Autodesk Fusion 360 part; units mm, degrees
(part 2 of 2)
sketch "Access Holes (Front)" plane through (-47, 0, 0) normal (1, 0, 0) x (0, 1, 0)
  line L0 (-30, 10) -> (30, 10)
  line L1 (30, 10) -> (30, 28)
  line L2 (30, 28) -> (-30, 28)
  line L3 (-30, 28) -> (-30, 10)
  line L4 (-18, 28) -> (-18, 10)
  line L5 (-9, 10) -> (-27, 10)
  line L6 (9, 28) -> (-7.0946, 28)
  line L7 (-7, 10) -> (9.0946, 10)
  line L8 (9, 28) -> (-7, 10) construction
  line L9 (-27, 10) -> (-9, 10)
  line L10 (-9, 10) -> (-9, 28)
  line L11 (-9, 28) -> (-27, 28)
  line L12 (-27, 28) -> (-27, 10)
  line L13 (-7, 10) -> (9, 10)
  line L14 (9, 10) -> (9, 28)
  line L15 (9, 28) -> (-7, 28)
  line L16 (-7, 28) -> (-7, 10)
  line L17 (11, 10) -> (27, 10)
  line L18 (27, 10) -> (27, 28)
  line L19 (27, 28) -> (11, 28)
  line L20 (11, 28) -> (11, 10)
  line L21 (30, 10) -> (-30, 10)
  line L22 (-13.2569, 0) -> (-15.855, 0)
  line L23 (-15.855, 0) -> (-18.4531, 0)
  line L24 (-18.4531, 0) -> (-15.855, 0)
  line L25 (-15.855, 0) -> (-13.2569, 0)
  line L26 (-15.4901, 0) -> (-12.892, 0)
  line L27 (-12.892, 0) -> (-10.2939, 0)
  line L28 (-10.2939, 0) -> (-12.892, 0)
  line L29 (-12.892, 0) -> (-15.4901, 0)
  line L30 (-7.0879, 0) -> (-9.686, 0)
  line L31 (-9.686, 0) -> (-12.2841, 0)
  line L32 (-12.2841, 0) -> (-9.686, 0)
  line L33 (-9.686, 0) -> (-7.0879, 0)
  line L34 (-21.6861, 0) -> (-19.088, 0)
  line L35 (-19.088, 0) -> (-16.4899, 0)
  line L36 (-16.4899, 0) -> (-19.088, 0)
  line L37 (-19.088, 0) -> (-21.6861, 0)
  line L38 (-15.4901, 0) -> (-12.892, 0)
  line L39 (-12.892, 0) -> (-10.2939, 0)
  line L40 (-10.2939, 0) -> (-12.892, 0)
  line L41 (-12.892, 0) -> (-15.4901, 0)
  line L42 (-9.2941, 0) -> (-6.696, 0)
  line L43 (-6.696, 0) -> (-4.0979, 0)
  line L44 (-4.0979, 0) -> (-6.696, 0)
  line L45 (-6.696, 0) -> (-9.2941, 0)
  line L46 (-0.5, 0) -> (2.0981, 0)
  line L47 (2.0981, 0) -> (-0.5, 0)
  line L48 (-0.5, 0) -> (-3.0981, 0)
  line L49 (-3.0981, 0) -> (-0.5, 0)
  line L50 (-9.2941, 0) -> (-6.696, 0)
  line L51 (-6.696, 0) -> (-4.0979, 0)
  line L52 (-4.0979, 0) -> (-6.696, 0)
  line L53 (-6.696, 0) -> (-9.2941, 0)
  line L54 (-7.0879, 0) -> (-9.686, 0)
  line L55 (-9.686, 0) -> (-12.2841, 0)
  line L56 (-12.2841, 0) -> (-9.686, 0)
  line L57 (-9.686, 0) -> (-7.0879, 0)
  line L58 (-0.9189, 0) -> (-3.517, 0)
  line L59 (-3.517, 0) -> (-6.1151, 0)
  line L60 (-6.1151, 0) -> (-3.517, 0)
  line L61 (-3.517, 0) -> (-0.9189, 0)
  line L62 (5.2501, 0) -> (2.652, 0)
  line L63 (2.652, 0) -> (0.0539, 0)
  line L64 (0.0539, 0) -> (2.652, 0)
  line L65 (2.652, 0) -> (5.2501, 0)
  line L66 (11.4191, 0) -> (8.821, 0)
  line L67 (8.821, 0) -> (6.2229, 0)
  line L68 (6.2229, 0) -> (8.821, 0)
  line L69 (8.821, 0) -> (11.4191, 0)
  line L70 (5.696, 0) -> (8.2941, 0)
  line L71 (8.2941, 0) -> (5.696, 0)
  line L72 (5.696, 0) -> (3.0979, 0)
  line L73 (3.0979, 0) -> (5.696, 0)
  line L74 (18.088, 0) -> (15.4899, 0)
  line L75 (15.4899, 0) -> (18.088, 0)
  line L76 (18.088, 0) -> (20.6861, 0)
  line L77 (20.6861, 0) -> (18.088, 0)
  line L78 (11.892, 0) -> (14.4901, 0)
  line L79 (14.4901, 0) -> (11.892, 0)
  line L80 (11.892, 0) -> (9.2939, 0)
  line L81 (9.2939, 0) -> (11.892, 0)
  line L82 (-0.5, 0) -> (2.0981, 0)
  line L83 (2.0981, 0) -> (-0.5, 0)
  line L84 (-0.5, 0) -> (-3.0981, 0)
  line L85 (-3.0981, 0) -> (-0.5, 0)
  line L86 (11.4191, 0) -> (8.821, 0)
  line L87 (8.821, 0) -> (6.2229, 0)
  line L88 (6.2229, 0) -> (8.821, 0)
  line L89 (8.821, 0) -> (11.4191, 0)
  line L90 (11.4191, 0) -> (8.821, 0)
  line L91 (8.821, 0) -> (6.2229, 0)
  line L92 (6.2229, 0) -> (8.821, 0)
  line L93 (8.821, 0) -> (11.4191, 0)
  line L94 (20.6861, 0) -> (18.088, 0)
  line L95 (18.088, 0) -> (15.4899, 0)
  line L96 (15.4899, 0) -> (18.088, 0)
  line L97 (18.088, 0) -> (20.6861, 0)
  line L98 (20.6861, 0) -> (18.088, 0)
  line L99 (18.088, 0) -> (15.4899, 0)
  line L100 (15.4899, 0) -> (18.088, 0)
  line L101 (18.088, 0) -> (20.6861, 0)
  line L102 (17.5881, 0) -> (14.99, 0)
  line L103 (14.99, 0) -> (12.3919, 0)
  line L104 (12.3919, 0) -> (14.99, 0)
  line L105 (14.99, 0) -> (17.5881, 0)
  line L106 (11.892, 0) -> (14.4901, 0)
  line L107 (14.4901, 0) -> (11.892, 0)
  line L108 (11.892, 0) -> (9.2939, 0)
  line L109 (9.2939, 0) -> (11.892, 0)
  line L110 (5.2501, 0) -> (2.652, 0)
  line L111 (2.652, 0) -> (0.0539, 0)
  line L112 (0.0539, 0) -> (2.652, 0)
  line L113 (2.652, 0) -> (5.2501, 0)
  line L114 (5.2501, 0) -> (2.652, 0)
  line L115 (2.652, 0) -> (0.0539, 0)
  line L116 (0.0539, 0) -> (2.652, 0)
  line L117 (2.652, 0) -> (5.2501, 0)
  line L118 (17.5881, 0) -> (14.99, 0)
  line L119 (14.99, 0) -> (12.3919, 0)
  line L120 (12.3919, 0) -> (14.99, 0)
  line L121 (14.99, 0) -> (17.5881, 0)
  line L122 (9.2939, 0) -> (11.892, 0)
  line L123 (11.892, 0) -> (14.4901, 0)
  line L124 (14.4901, 0) -> (11.892, 0)
  line L125 (11.892, 0) -> (9.2939, 0)
  line L126 (11.4191, 0) -> (8.821, 0)
  line L127 (8.821, 0) -> (6.2229, 0)
  line L128 (6.2229, 0) -> (8.821, 0)
  line L129 (8.821, 0) -> (11.4191, 0)
  line L130 (5.2501, 0) -> (2.652, 0)
  line L131 (2.652, 0) -> (0.0539, 0)
  line L132 (0.0539, 0) -> (2.652, 0)
  line L133 (2.652, 0) -> (5.2501, 0)
  line L134 (-0.9189, 0) -> (-3.517, 0)
  line L135 (-3.517, 0) -> (-6.1151, 0)
  line L136 (-6.1151, 0) -> (-3.517, 0)
  line L137 (-3.517, 0) -> (-0.9189, 0)
  line L138 (-7.0879, 0) -> (-9.686, 0)
  line L139 (-9.686, 0) -> (-12.2841, 0)
  line L140 (-12.2841, 0) -> (-9.686, 0)
  line L141 (-9.686, 0) -> (-7.0879, 0)
  line L142 (3.0979, 0) -> (5.696, 0)
  line L143 (5.696, 0) -> (8.2941, 0)
  line L144 (8.2941, 0) -> (5.696, 0)
  line L145 (5.696, 0) -> (3.0979, 0)
  line L146 (-0.9189, 0) -> (-3.517, 0)
  line L147 (-3.517, 0) -> (-6.1151, 0)
  line L148 (-6.1151, 0) -> (-3.517, 0)
  line L149 (-3.517, 0) -> (-0.9189, 0)
  line L150 (-9.2941, 0) -> (-6.696, 0)
  line L151 (-6.696, 0) -> (-4.0979, 0)
  line L152 (-4.0979, 0) -> (-6.696, 0)
  line L153 (-6.696, 0) -> (-9.2941, 0)
  line L154 (-15.4901, 0) -> (-12.892, 0)
  line L155 (-12.892, 0) -> (-10.2939, 0)
  line L156 (-10.2939, 0) -> (-12.892, 0)
  line L157 (-12.892, 0) -> (-15.4901, 0)
  line L158 (-21.6861, 0) -> (-19.088, 0)
  line L159 (-19.088, 0) -> (-16.4899, 0)
  line L160 (-16.4899, 0) -> (-19.088, 0)
  line L161 (-19.088, 0) -> (-21.6861, 0)
  line L162 (-15.4901, 0) -> (-12.892, 0)
  line L163 (-12.892, 0) -> (-10.2939, 0)
  line L164 (-10.2939, 0) -> (-12.892, 0)
  line L165 (-12.892, 0) -> (-15.4901, 0)
  line L166 (-15.4901, 0) -> (-12.892, 0)
  line L167 (-12.892, 0) -> (-10.2939, 0)
  line L168 (-10.2939, 0) -> (-12.892, 0)
  line L169 (-12.892, 0) -> (-15.4901, 0)
  line L170 (-21.6861, 0) -> (-19.088, 0)
  line L171 (-19.088, 0) -> (-16.4899, 0)
  line L172 (-16.4899, 0) -> (-19.088, 0)
  line L173 (-19.088, 0) -> (-21.6861, 0)
  line L174 (-21.6861, 0) -> (-19.088, 0)
  line L175 (-19.088, 0) -> (-16.4899, 0)
  line L176 (-16.4899, 0) -> (-19.088, 0)
  line L177 (-19.088, 0) -> (-21.6861, 0)
  line L178 (-21.6861, 0) -> (-19.088, 0)
  line L179 (-19.088, 0) -> (-16.4899, 0)
  line L180 (-16.4899, 0) -> (-19.088, 0)
  line L181 (-19.088, 0) -> (-21.6861, 0)
  line L182 (-13.2569, 0) -> (-15.855, 0)
  line L183 (-15.855, 0) -> (-18.4531, 0)
  line L184 (-18.4531, 0) -> (-15.855, 0)
  line L185 (-15.855, 0) -> (-13.2569, 0)
  line L186 (-9.2941, 0) -> (-6.696, 0)
  line L187 (-6.696, 0) -> (-4.0979, 0)
  line L188 (-4.0979, 0) -> (-6.696, 0)
  line L189 (-6.696, 0) -> (-9.2941, 0)
  line L190 (-15.4901, 0) -> (-12.892, 0)
  line L191 (-12.892, 0) -> (-10.2939, 0)
  line L192 (-10.2939, 0) -> (-12.892, 0)
  line L193 (-12.892, 0) -> (-15.4901, 0)
  line L194 (-13.2569, 0) -> (-15.855, 0)
  line L195 (-15.855, 0) -> (-18.4531, 0)
  line L196 (-18.4531, 0) -> (-15.855, 0)
  line L197 (-15.855, 0) -> (-13.2569, 0)
  line L198 (-7.0879, 0) -> (-9.686, 0)
  line L199 (-9.686, 0) -> (-12.2841, 0)
  line L200 (-12.2841, 0) -> (-9.686, 0)
  line L201 (-9.686, 0) -> (-7.0879, 0)
  line L202 (-0.9189, 0) -> (-3.517, 0)
  line L203 (-3.517, 0) -> (-6.1151, 0)
  line L204 (-6.1151, 0) -> (-3.517, 0)
  line L205 (-3.517, 0) -> (-0.9189, 0)
  line L206 (5.2501, 0) -> (2.652, 0)
  line L207 (2.652, 0) -> (0.0539, 0)
  line L208 (0.0539, 0) -> (2.652, 0)
  line L209 (2.652, 0) -> (5.2501, 0)
  line L210 (-0.9189, 0) -> (-3.517, 0)
  line L211 (-3.517, 0) -> (-6.1151, 0)
  line L212 (-6.1151, 0) -> (-3.517, 0)
  line L213 (-3.517, 0) -> (-0.9189, 0)
  line L214 (-9.2941, 0) -> (-6.696, 0)
  line L215 (-6.696, 0) -> (-4.0979, 0)
  line L216 (-4.0979, 0) -> (-6.696, 0)
  line L217 (-6.696, 0) -> (-9.2941, 0)
  line L218 (-0.5, 0) -> (2.0981, 0)
  line L219 (2.0981, 0) -> (-0.5, 0)
  line L220 (-0.5, 0) -> (-3.0981, 0)
  line L221 (-3.0981, 0) -> (-0.5, 0)
  line L222 (5.696, 0) -> (8.2941, 0)
  line L223 (8.2941, 0) -> (5.696, 0)
  line L224 (5.696, 0) -> (3.0979, 0)
  line L225 (3.0979, 0) -> (5.696, 0)
  line L226 (11.892, 0) -> (14.4901, 0)
  line L227 (14.4901, 0) -> (11.892, 0)
  line L228 (11.892, 0) -> (9.2939, 0)
  line L229 (9.2939, 0) -> (11.892, 0)
  line L230 (12.3919, 0) -> (14.99, 0)
  line L231 (14.99, 0) -> (17.5881, 0)
  line L232 (17.5881, 0) -> (14.99, 0)
  line L233 (14.99, 0) -> (12.3919, 0)
  line L234 (17.5881, 0) -> (14.99, 0)
  line L235 (14.99, 0) -> (12.3919, 0)
  line L236 (12.3919, 0) -> (14.99, 0)
  line L237 (14.99, 0) -> (17.5881, 0)
  line L238 (5.696, 0) -> (8.2941, 0)
  line L239 (8.2941, 0) -> (5.696, 0)
  line L240 (5.696, 0) -> (3.0979, 0)
  line L241 (3.0979, 0) -> (5.696, 0)
  line L242 (17.5881, 0) -> (14.99, 0)
  line L243 (14.99, 0) -> (12.3919, 0)
  line L244 (12.3919, 0) -> (14.99, 0)
  line L245 (14.99, 0) -> (17.5881, 0)
  line L246 (17.5881, 0) -> (14.99, 0)
  line L247 (14.99, 0) -> (12.3919, 0)
  line L248 (12.3919, 0) -> (14.99, 0)
  line L249 (14.99, 0) -> (17.5881, 0)
  line L250 (20.6861, 0) -> (18.088, 0)
  line L251 (18.088, 0) -> (15.4899, 0)
  line L252 (15.4899, 0) -> (18.088, 0)
  line L253 (18.088, 0) -> (20.6861, 0)
  line L254 (20.6861, 0) -> (18.088, 0)
  line L255 (18.088, 0) -> (15.4899, 0)
  line L256 (15.4899, 0) -> (18.088, 0)
  line L257 (18.088, 0) -> (20.6861, 0)
  line L258 (11.892, 0) -> (14.4901, 0)
  line L259 (14.4901, 0) -> (11.892, 0)
  line L260 (11.892, 0) -> (9.2939, 0)
  line L261 (9.2939, 0) -> (11.892, 0)
  line L262 (5.696, 0) -> (8.2941, 0)
  line L263 (8.2941, 0) -> (5.696, 0)
  line L264 (5.696, 0) -> (3.0979, 0)
  line L265 (3.0979, 0) -> (5.696, 0)
  line L266 (11.892, 0) -> (14.4901, 0)
  line L267 (14.4901, 0) -> (11.892, 0)
  line L268 (11.892, 0) -> (9.2939, 0)
  line L269 (9.2939, 0) -> (11.892, 0)
  line L270 (11.4191, 0) -> (8.821, 0)
  line L271 (8.821, 0) -> (6.2229, 0)
  line L272 (6.2229, 0) -> (8.821, 0)
  line L273 (8.821, 0) -> (11.4191, 0)
  line L274 (20.6861, 0) -> (18.088, 0)
  line L275 (18.088, 0) -> (15.4899, 0)
  line L276 (15.4899, 0) -> (18.088, 0)
  line L277 (18.088, 0) -> (20.6861, 0)
  line L278 (11.4191, 0) -> (8.821, 0)
  line L279 (8.821, 0) -> (6.2229, 0)
  line L280 (6.2229, 0) -> (8.821, 0)
  line L281 (8.821, 0) -> (11.4191, 0)
  line L282 (5.2501, 0) -> (2.652, 0)
  line L283 (2.652, 0) -> (0.0539, 0)
  line L284 (0.0539, 0) -> (2.652, 0)
  line L285 (2.652, 0) -> (5.2501, 0)
  line L286 (5.696, 0) -> (8.2941, 0)
  line L287 (8.2941, 0) -> (5.696, 0)
  line L288 (5.696, 0) -> (3.0979, 0)
  line L289 (3.0979, 0) -> (5.696, 0)
  line L290 (-0.5, 0) -> (2.0981, 0)
  line L291 (2.0981, 0) -> (-0.5, 0)
  line L292 (-0.5, 0) -> (-3.0981, 0)
  line L293 (-3.0981, 0) -> (-0.5, 0)
  line L294 (-9.2941, 0) -> (-6.696, 0)
  line L295 (-6.696, 0) -> (-4.0979, 0)
  line L296 (-4.0979, 0) -> (-6.696, 0)
  line L297 (-6.696, 0) -> (-9.2941, 0)
  line L298 (-3.0981, 0) -> (-0.5, 0)
  line L299 (-0.5, 0) -> (2.0981, 0)
  line L300 (2.0981, 0) -> (-0.5, 0)
  line L301 (-0.5, 0) -> (-3.0981, 0)
  line L302 (-0.5, 0) -> (2.0981, 0)
  line L303 (2.0981, 0) -> (-0.5, 0)
  line L304 (-0.5, 0) -> (-3.0981, 0)
  line L305 (-3.0981, 0) -> (-0.5, 0)
  line L306 (-0.9189, 0) -> (-3.517, 0)
  line L307 (-3.517, 0) -> (-6.1151, 0)
  line L308 (-6.1151, 0) -> (-3.517, 0)
  line L309 (-3.517, 0) -> (-0.9189, 0)
  line L310 (-7.0879, 0) -> (-9.686, 0)
  line L311 (-9.686, 0) -> (-12.2841, 0)
  line L312 (-12.2841, 0) -> (-9.686, 0)
  line L313 (-9.686, 0) -> (-7.0879, 0)
  line L314 (-13.2569, 0) -> (-15.855, 0)
  line L315 (-15.855, 0) -> (-18.4531, 0)
  line L316 (-18.4531, 0) -> (-15.855, 0)
  line L317 (-15.855, 0) -> (-13.2569, 0)
  line L318 (-7.0879, 0) -> (-9.686, 0)
  line L319 (-9.686, 0) -> (-12.2841, 0)
  line L320 (-12.2841, 0) -> (-9.686, 0)
  line L321 (-9.686, 0) -> (-7.0879, 0)
  line L322 (-21.6861, 0) -> (-19.088, 0)
  line L323 (-19.088, 0) -> (-16.4899, 0)
  line L324 (-16.4899, 0) -> (-19.088, 0)
  line L325 (-19.088, 0) -> (-21.6861, 0)
  line L326 (-13.2569, 0) -> (-15.855, 0)
  line L327 (-15.855, 0) -> (-18.4531, 0)
  line L328 (-18.4531, 0) -> (-15.855, 0)
  line L329 (-15.855, 0) -> (-13.2569, 0)
  line L330 (-13.2569, 0) -> (-15.855, 0)
  line L331 (-15.855, 0) -> (-18.4531, 0)
  line L332 (-18.4531, 0) -> (-15.855, 0)
  line L333 (-15.855, 0) -> (-13.2569, 0)
  line L334 (55, 0) -> (-55, 0)
  line L335 (-41, 0) -> (-49, 0)
  line L336 (49, 0) -> (41, 0)
  line L337 (4, 0) -> (-4, 0)
  line L338 (-9.2941, 0) -> (-6.696, 0)
  line L339 (-6.696, 0) -> (-4.0979, 0)
  line L340 (-4.0979, 0) -> (-6.696, 0)
  line L341 (-6.696, 0) -> (-9.2941, 0)
  line L342 (20.6861, 0) -> (18.088, 0)
  line L343 (18.088, 0) -> (15.4899, 0)
  line L344 (15.4899, 0) -> (18.088, 0)
  line L345 (18.088, 0) -> (20.6861, 0)
  line L346 (-3.0981, 0) -> (-0.5, 0)
  line L347 (-0.5, 0) -> (2.0981, 0)
  line L348 (2.0981, 0) -> (-0.5, 0)
  line L349 (-0.5, 0) -> (-3.0981, 0)
  line L350 (-15.4901, 0) -> (-12.892, 0)
  line L351 (-12.892, 0) -> (-10.2939, 0)
  line L352 (-10.2939, 0) -> (-12.892, 0)
  line L353 (-12.892, 0) -> (-15.4901, 0)
  line L354 (9.2939, 0) -> (11.892, 0)
  line L355 (11.892, 0) -> (14.4901, 0)
  line L356 (14.4901, 0) -> (11.892, 0)
  line L357 (11.892, 0) -> (9.2939, 0)
  line L358 (3.0979, 0) -> (5.696, 0)
  line L359 (5.696, 0) -> (8.2941, 0)
  line L360 (8.2941, 0) -> (5.696, 0)
  line L361 (5.696, 0) -> (3.0979, 0)
  line L362 (-21.6861, 0) -> (-19.088, 0)
  line L363 (-19.088, 0) -> (-16.4899, 0)
  line L364 (-16.4899, 0) -> (-19.088, 0)
  line L365 (-19.088, 0) -> (-21.6861, 0)
  point P0 (-18, 19)
  point P1 (-18, 19)
  point P2 (-18, 19)
  point P3 (1, 19)
  point P4 (1, 19)
  point P5 (19, 19)
  point P6 (0, 28)
  dimension "d108" = 18
  dimension "d112" = 11
  dimension "d113" = 8
  dimension "d114" = 8
  dimension "d115" = 9
  dimension "d116" = 8
  dimension "d117" = 8
  dimension "d152" = 2
  dimension "d153" = 2
  constraint coincident P2 P1
  constraint coincident L2 L4.start
  constraint perpendicular L2 L4
  constraint coincident L0 L4.end
  constraint midpoint P2 L4
  constraint horizontal P2 P4
  constraint horizontal L6
  constraint parallel L6 L7
  constraint coincident L8 P4
  constraint coincident L2 L6.start
  constraint coincident P4 P3
  constraint horizontal L9
  constraint vertical L10
  constraint horizontal L11
  constraint vertical L12
  constraint coincident L5.start L10
  constraint horizontal L13
  constraint vertical L14
  constraint horizontal L15
  constraint vertical L16
  constraint horizontal P4 P5
  constraint horizontal L17
  constraint vertical L18
  constraint horizontal L19
  constraint vertical L20
  constraint collinear L7 L21
  constraint collinear L0 L17
  constraint equal L14 L20
  constraint collinear L2 L11
  constraint equal L10 L16
  constraint midpoint L2 P6
  measures "d108" distance of L5.start L5.end
  measures "d112" distance of L1 P5
  measures "d113" distance of P4 L16
  measures "d114" distance of P4 L14
  measures "d115" distance of P2 L10
  measures "d116" distance of P5 L20
  measures "d117" distance of P5 L18
  measures "d152" distance of L14 L20
  measures "d153" distance of L10 L16
extrude "Extrude6" cut sketch "Access Holes (Front)" against normal through all contours L0 L2 L4 L5 L9 L11 L12 L21 | L0 L2 L4 L5 L9 L10 L11 L21 | L0 L2 L6 L7 L13 L14 L15 L16 L21 | L0 L2 L17 L18 L19 L20 L21
sketch "Soft Connectors" plane through (0, 0, 28) normal (0, 0, 1) x (-1, 0, 0)
  line L0 (47, 27) -> (53.5817, 27)
  arc A0 (53.5817, 27) -> (53.5817, -27) centre (0, 0) ccw
  line L1 (53.5817, -27) -> (47, -27)
  line L2 (47, -27) -> (47, -30)
  line L3 (47, -30) -> (-47, -30)
  line L4 (-47, -30) -> (-47, 30)
  line L5 (-47, 30) -> (47, 30)
  line L6 (47, 30) -> (47, 27)
  line L7 (-20, -45) -> (20, -45)
  line L8 (20, -45) -> (20, 45)
  line L9 (20, 45) -> (-20, 45)
  line L10 (-20, 45) -> (-20, -45)
  line L11 (-20, -45) -> (20, 45) construction
  line L12 (20, -45) -> (-20, 45) construction
  circle A1 centre (-50, 0) radius 1.666
  circle A2 centre (21.7945, 45) radius 1.666
  circle A3 centre (21.7945, -45) radius 1.666
  dimension "d121" = 40
  dimension "d122" = 90
  constraint horizontal L7
  constraint perpendicular L7 L8
  constraint parallel L7 L9
  constraint parallel L8 L10
  constraint coincident L11 A0.centre
  constraint coincident L12 A0.centre
  constraint coincident A0.centre origin
  measures "d121" distance of L7.start L7.end
  measures "d122" distance of L7.start L9.end
hole "Hole5" at (20, 45, 28) at (20, -45, 28) direction (0, 0, -1) diameter 5 depth 5 tip angle 180
sketch "Slots" plane through (0, 0, 28) normal (0, 0, 1) x (-1, 0, 0)
  circle A0 centre (-20, -45) radius 2.5
  circle A1 centre (-20, 45) radius 2.5
  line L0 (47, 27) -> (53.5817, 27)
  arc A2 (53.5817, 27) -> (53.5817, -27) centre (0, 0) ccw
  line L1 (53.5817, -27) -> (47, -27)
  line L2 (47, -27) -> (47, -30)
  line L3 (47, -30) -> (-47, -30)
  line L4 (-47, -30) -> (-47, 30)
  line L5 (-47, 30) -> (47, 30)
  line L6 (47, 30) -> (47, 27)
  line L7 (2.131, -32) -> (-7.869, -32)
  line L8 (-7.869, -32) -> (-7.869, -30)
  line L9 (-7.869, -30) -> (2.131, -30)
  line L10 (2.131, -30) -> (2.131, -32)
  line L11 (2.131, -32) -> (-7.869, -30) construction
  line L12 (-7.869, -32) -> (2.131, -30) construction
  line L13 (-7.869, -30) -> (2.131, -30)
  line L14 (-11, -32) -> (-21, -32)
  line L15 (-21, -32) -> (-21, -30)
  line L16 (-21, -30) -> (-11, -30)
  line L17 (-11, -30) -> (-11, -32)
  line L18 (-11, -32) -> (-21, -30) construction
  line L19 (-21, -32) -> (-11, -30) construction
  line L20 (-11, -30) -> (-21, -30)
  line L21 (-25.8, -32) -> (-35.8, -32)
  line L22 (-35.8, -32) -> (-35.8, -30)
  line L23 (-35.8, -30) -> (-25.8, -30)
  line L24 (-25.8, -30) -> (-25.8, -32)
  line L25 (-25.8, -32) -> (-35.8, -30) construction
  line L26 (-35.8, -32) -> (-25.8, -30) construction
  line L27 (-35.8, -30) -> (-25.8, -30)
  line L28 (6.1122, -50) -> (16.1122, -50)
  line L29 (16.1122, -50) -> (16.1122, -30)
  line L30 (16.1122, -30) -> (6.1122, -30)
  line L31 (6.1122, -30) -> (6.1122, -50)
  circle A3 centre (-50, 0) radius 1.666
  circle A4 centre (21.7945, 45) radius 1.666
  circle A5 centre (21.7945, -45) radius 1.666
  line L32 (2.131, -30) -> (-35.8, -30)
  line L33 (-35.8, -30) -> (-35.8, -32)
  line L34 (-35.8, -32) -> (2.131, -32)
  line L35 (2.131, -32) -> (2.131, -30)
  point P0 (-2.5, -30)
  point P1 (-2.869, -31)
  point P2 (-16, -31)
  point P3 (-16, -30)
  point P4 (-30.8, -31)
  point P5 (-30.8, -30)
  point P6 (11.131, -31)
  point P7 (11.131, -31)
  dimension "d130" = 2
  dimension "d131" = 2
  dimension "d132" = 2
  dimension "d135" = 14
  dimension "d136" = 10
  dimension "d137" = 20
  constraint horizontal L7
  constraint perpendicular L7 L8
  constraint parallel L7 L9
  constraint parallel L8 L10
  constraint coincident L11 P1
  constraint coincident L12 P1
  constraint equal L9 L13
  constraint collinear L9 L13
  constraint horizontal L14
  constraint perpendicular L14 L15
  constraint parallel L14 L16
  constraint parallel L15 L17
  constraint coincident L18 P2
  constraint coincident L19 P2
  constraint vertical P2 P3
  constraint equal L16 L20
  constraint collinear L16 L20
  constraint horizontal L21
  constraint perpendicular L21 L22
  constraint parallel L21 L23
  constraint parallel L22 L24
  constraint coincident L25 P4
  constraint coincident L26 P4
  constraint equal L23 L27
  constraint vertical P4 P5
  constraint collinear L23 L27
  constraint coincident L9.end L10.start
  constraint horizontal P1 P7
  constraint perpendicular L28 L29
  constraint parallel L28 L30
  constraint coincident P7 P6
  constraint collinear L3 L30
  constraint equal L29 L31
  constraint horizontal L32
  constraint vertical L33
  constraint horizontal L34
  constraint vertical L35
  measures "d130" distance of L7.start L9.end
  measures "d131" distance of L14.start L16.end
  measures "d132" distance of L21.start L23.end
  measures "d135" distance of P1 P7
  measures "d136" distance of L28.start L28.end
  measures "d137" distance of L28.start L30.end
extrude "Extrude7" cut sketch "Slots" against normal up to surface (18 mm away) contours L3 L21 L22 L23 L24 L27 L32 L33 L34 | L3 L28 L29 L30 L31 | L3 L15 L24 L32 L34 | L3 L14 L15 L16 L17 L20 L32 L34 | L3 L7 L8 L9 L10 L13 L32 L34 L35 | L3 L8 L17 L32 L34
other "Base Mesh Feature2"
other "Modify3"
other "Modify4"
other "Modify5"
fillet "Fillet1" radius 4 6 edges at (-50.2909, -27, 10) (-53.2951, -7, 10) (-53.1606, 9, 10) (-50.2909, 27, 10) (-52.9915, 11, 10) (-53.1606, -9, 10)
equation "d61 = 7.7 mm + 3.5 mm + 5 mm"
equation "d79 = 9.5 mm + 1.5 mm"
equation "d81 = 9.412 mm + 2.5 mm"
equation "d86 = 5.196 mm + 1 mm"
equation "d97 = 5.169 mm + 1 mm"
